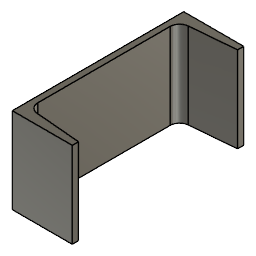
C-200×70×7.0×10 (Autodesk Fusion 360 design; units mm, degrees)
Autodesk Fusion 360 part; units mm, degrees
note: some values were not read from the file. Set by a fixed rule: which sketch regions a step uses.
sketch "スケッチ1" plane through (0, 0, 0) normal (0, 0, 1) x (1, 0, 0)
  line L0 (7, 177.1645) -> (7, 22.8355)
  line L1 (0, 200) -> (0, 0)
  line L2 (0, 0) -> (70, 0)
  line L3 (70, 7.2441) -> (70, 0)
  line L4 (17.0413, 11.8774) -> (70, 7.2441)
  line L5 (70, 192.7559) -> (17.0413, 188.1226)
  line L6 (0, 200) -> (70, 200)
  line L7 (70, 200) -> (70, 192.7559)
  arc A0 (7, 22.8355) -> (17.0413, 11.8774) centre (18, 22.8355) ccw
  arc A1 (17.0413, 188.1226) -> (7, 177.1645) centre (18, 177.1645) ccw
extrude "押し出し1" add sketch "スケッチ1" along normal blind 100
